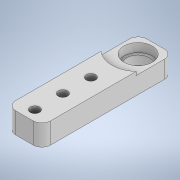
# Autodesk Inventor part: top support
Saved by Autodesk Inventor 2022 (Build 260153000, 153)
## iProperties
Created: 2022-03-10
Part Number: top support
Material: Genérico
Document SubType Name: Modeling
Designer: JK
Density: 1 g/cm^3
Appearance: Valor por defecto
Author: JK
Autodesk Inventor part; units mm, degrees
ref_plane "YZ Plane" through (0, 0, 0) normal (1, 0, 0) x (0, 1, 0)
ref_plane "XZ Plane" through (0, 0, 0) normal (0, 1, 0) x (-1, 0, 0)
ref_plane "XY Plane" through (0, 0, 0) normal (0, 0, 1) x (1, 0, 0)
sketch "Boceto1" plane through (0, 0, 0) normal (0, 1, 0) x (-1, 0, 0)
  line L0 (-10, 37.5) -> (10, 37.5)
  line L1 (10, 37.5) -> (10, -37.5)
  line L2 (10, -37.5) -> (-10, -37.5)
  line L3 (-10, -37.5) -> (-10, 37.5)
  line L4 (-10, 37.5) -> (10, -37.5) construction
  line L5 (10, 37.5) -> (-10, -37.5) construction
  circle A0 centre (0, -27.5) radius 8.125
  point P0 (0, 0)
  point P1 (5.4787, -34.25)
  point P2 (-5.4787, -34.25)
  dimension "d0" = 20
  dimension "d23" = 65
  dimension "d24" = 10
  dimension "d25" = 16.25
  constraints: 12 end point, 2 midpoint, 2 parallel, 1 centre point, 1 horizontal, 1 perpendicular
  measures "d0" distance of L0.start L0.end
  measures "d23" distance from line of L0 A0.centre
  measures "d24" distance from line of L2 A0.centre
  measures "d25" diameter of A0
extrude "Extrusión1" add sketch "Boceto1" along normal blind 12 contours L0 L1 L2 L3 | A0
sketch "Boceto5" plane through (0, 12, 0) normal (0, 1, 0) x (1, 0, 0)
  circle A0 centre (0, 27.5) radius 8.125
  line L0 (10, 37.5) -> (-10, 37.5) projected
  line L1 (-10, -37.5) -> (10, -37.5) projected
  point P0 (0, 0)
  dimension "d26" = 16.25
  dimension "d36" = 65
  constraints: 1 centre point
  measures "d26" diameter of A0
  measures "d36" distance from line of L1 A0.centre
extrude "Extrusión5" cut sketch "Boceto5" against normal blind 7
sketch "Boceto6" plane through (0, 5, -27.5) normal (0, 1, 0) x (1, 0, 0)
  circle A0 centre (0, 0) radius 6.5
  point P0 (0, -27.5)
  dimension "d30" = 13
  constraints: 1 centre point
  measures "d30" diameter of A0
extrude "Extrusión6" cut sketch "Boceto6" against normal through all
sketch "Boceto7" plane through (0, 12, 0) normal (0, 1, 0) x (1, 0, 0)
  circle A0 centre (0, 27.5) radius 8.125 projected
  circle A1 centre (0, 27.5) radius 15
  point P0 (0, 0)
  dimension "d33" = 30
  constraints: 1 centre point, 1 coincident
  measures "d33" diameter of A1
extrude "Extrusión7" cut sketch "Boceto7" against normal blind 2
fillet "Empalme5" radius 5 2 edges at (-10, 6, 37.5) (10, 6, 37.5)
fillet "Empalme6" radius 5 2 edges at (10, 5, -37.5) (-10, 5, -37.5)
sketch "Boceto8" plane through (0, 0, 0) normal (0, -1, 0) x (1, 0, 0)
  circle A0 centre (0, 31.5) radius 2.7
  circle A1 centre (0, 15.5) radius 2.7
  line L0 (-5, 37.5) -> (5, 37.5) projected
  circle A2 centre (0, -0.5) radius 2.7
  point P0 (0, 0)
  dimension "d39" = 5.4
  dimension "d40" = 6
  dimension "d41" = 16
  dimension "d47" = 16
  constraints: 3 centre point, 2 equal radius
  measures "d39" diameter of A0
  measures "d40" distance from line of L0 A0.centre
  measures "d41" distance of A1.centre A0.centre
  measures "d47" distance of A2.centre A1.centre
extrude "Extrusión8" cut sketch "Boceto8" against normal through all
sketch "Boceto9" plane through (0, 0, 0) normal (0, -1, 0) x (1, 0, 0)
  circle A0 centre (0, 31.5) radius 2.7 projected
  circle A1 centre (0, 31.5) radius 4.65
  circle A2 centre (0, 15.5) radius 2.7 projected
  circle A3 centre (0, 15.5) radius 4.65
  circle A4 centre (0, -0.5) radius 2.7 projected
  circle A5 centre (0, -0.5) radius 4.65
  point P0 (0, 0)
  dimension "d44" = 9.3
  constraints: 3 centre point, 3 coincident, 2 equal radius
  measures "d44" diameter of A1
extrude "Extrusión9" cut sketch "Boceto9" against normal blind 2 contours A0 | A1 | A2 | A3 | A4 | A5
sketch "Boceto2" plane through (0, 12, 0) normal (0, 1, 0) x (1, 0, 0)
  line L0 (10, 37.5) -> (-10, 37.5) projected
  line L1 (-10, 37.5) -> (5, 37.5)
  line L2 (5, 37.5) -> (5, 77.5)
  line L3 (5, 77.5) -> (-5, 77.5)
  line L4 (-5, 77.5) -> (-5, 37.5)
  circle A0 centre (0, 70) radius 2.7
  line L5 (10, -37.5) -> (10, 37.5) projected
  line L6 (10, 37.5) -> (-10, 37.5) projected
  point P0 (0, 0)
  point P1 (5, 20)
  point P2 (-5, 20)
  dimension "d4" = 5.4
  dimension "d5" = 7.5
  dimension "d19" = 40
  dimension "d20" = 5
  dimension "d21" = 5
  dimension "d22" = 5
  constraints: 8 end point, 2 parallel, 1 centre point, 1 horizontal, 1 perpendicular, 1 point on line
  measures "d4" diameter of A0
  measures "d5" distance from line of L3 A0.centre
  measures "d19" distance between parallel lines of L0 L3
  measures "d20" distance from line of A0.centre L4
  measures "d21" distance from line of L2 A0.centre
  measures "d22" distance between parallel lines of L5 L2
sketch "Boceto3" plane through (0, 10.5, 0) normal (0, -1, 0) x (1, 0, 0)
  circle A0 centre (0, -52.5) radius 2.7 projected
  circle A1 centre (0, -52.5) radius 5
  line L0 (5, -60) -> (5, -20) projected
  point P0 (0, 0)
  constraints: 1 centre point, 1 coincident, 1 tangent
sketch "Boceto4" plane through (0, 0, 0) normal (0, -1, 0) x (1, 0, 0)
  circle A0 centre (0, -8) radius 2.7
  circle A1 centre (0, 8) radius 2.7
  point P0 (0, 0)
  dimension "d13" = 5.4
  dimension "d14" = 8
  dimension "d15" = 8
  constraints: 2 centre point, 1 equal radius
  measures "d13" diameter of A1
  measures "d14" distance of A1.centre point (0, 0)
  measures "d15" distance of A0.centre point (0, 0)
